Baseplate_V2_v4 (Autodesk Fusion 360 design; units mm, degrees)
Autodesk Fusion 360 part; units mm, degrees
sketch "Esquisse2" plane through (0, 0, 0) normal (0, 0, 1) x (1, 0, 0)
  line L0 (160, 106.25) -> (-160, 106.25)
  line L1 (-160, 106.25) -> (-160, -106.25)
  line L2 (160, -106.25) -> (160, 106.25)
  line L3 (160, 106.25) -> (-160, -106.25) construction
  line L4 (-160, 106.25) -> (160, -106.25) construction
  line L5 (0, 0) -> (65, 0) construction
  line L6 (95, 45) -> (65, 45)
  line L7 (65, 45) -> (65, -45)
  line L8 (65, -45) -> (95, -45)
  line L9 (95, -45) -> (95, 45)
  line L10 (95, 45) -> (65, -45) construction
  line L11 (65, 45) -> (95, -45) construction
  line L12 (110, 45) -> (95, 45)
  line L13 (95, 45) -> (95, -45)
  line L14 (95, -45) -> (110, -45)
  line L15 (110, -45) -> (110, 45)
  line L16 (110, 45) -> (95, -45) construction
  line L17 (95, 45) -> (110, -45) construction
  circle A0 centre (150, 96.25) radius 2.5
  line L18 (0, 2.5) -> (0, 20)
  circle A1 centre (-150, 96.25) radius 2.5
  circle A2 centre (150, -96.25) radius 2.5
  circle A3 centre (-150, -96.25) radius 2.5
  circle A4 centre (0, 86.25) radius 12.5
  circle A5 centre (115, -106.25) radius 12.5
  line L19 (0, 1.75) -> (0, 22.5)
  circle A6 centre (-115, -106.25) radius 12.5
  arc A7 (-131.5, -106.25) -> (-98.5, -106.25) centre (-115, -106.25) ccw
  line L20 (-160, -106.25) -> (-131.5, -106.25)
  arc A8 (98.5, -106.25) -> (131.5, -106.25) centre (115, -106.25) ccw
  line L21 (-98.5, -106.25) -> (98.5, -106.25)
  line L22 (131.5, -106.25) -> (160, -106.25)
  line L23 (-65, 45) -> (-65, -45)
  line L24 (-95, 45) -> (-65, 45)
  line L25 (-110, 45) -> (-95, 45)
  line L26 (-110, -45) -> (-110, 45)
  line L27 (-95, -45) -> (-110, -45)
  line L28 (-65, -45) -> (-95, -45)
  line L29 (-155, 70) -> (-150, 70)
  line L30 (-150, 70) -> (-150, 30)
  line L31 (-150, 30) -> (-155, 30)
  line L32 (-155, 30) -> (-155, 70)
  line L33 (-155, -30) -> (-155, -70)
  line L34 (-150, -30) -> (-155, -30)
  line L35 (-150, -70) -> (-150, -30)
  line L36 (-155, -70) -> (-150, -70)
  line L37 (150, -70) -> (150, -30)
  line L38 (155, -70) -> (150, -70)
  line L39 (155, -30) -> (155, -70)
  line L40 (150, -30) -> (155, -30)
  line L41 (155, 30) -> (155, 70)
  line L42 (155, 70) -> (150, 70)
  line L43 (150, 70) -> (150, 30)
  line L44 (150, 30) -> (155, 30)
  point P0 (80, 0)
  point P1 (102.5, 0)
  dimension "d39" = 212.5
  dimension "d40" = 65
  dimension "d41" = 50
  dimension "d42" = 30
  dimension "d43" = 15
  dimension "d44" = 90
  dimension "d45" = 90
  dimension "d46" = 5
  dimension "d47" = 10
  dimension "d48" = 10
  dimension "d49" = 25
  dimension "d50" = 20
  dimension "d51" = 25
  dimension "d52" = 45
  dimension "d54" = 4
  dimension "d56" = 4
  dimension "d57" = 28.5
  dimension "d58" = 5
  dimension "d59" = 40
  dimension "d60" = 5
  dimension "d61" = 30
  constraint horizontal L0
  constraint perpendicular L0 L1
  constraint parallel L0 L20
  constraint parallel L1 L2
  constraint coincident L3 L5.start
  constraint coincident L4 L5.start
  constraint coincident L5.start origin
  constraint horizontal L5
  constraint horizontal L6
  constraint perpendicular L6 L7
  constraint parallel L6 L8
  constraint parallel L7 L9
  constraint coincident L10 P0
  constraint coincident L11 P0
  constraint horizontal L12
  constraint perpendicular L12 L13
  constraint parallel L12 L14
  constraint parallel L13 L15
  constraint coincident L16 P1
  constraint coincident L17 P1
  constraint collinear L9 L13
  constraint coincident L5.end L7
  constraint coincident L5 P0
  constraint coincident L5 P1
  constraint symmetric A0 L18 A1
  constraint symmetric L5 A0 A2
  constraint symmetric L5 A1 A3
  constraint coincident A5.centre L20
  constraint coincident A4.centre L19
  constraint symmetric A5 L19 A6
  constraint concentric A6 A7
  constraint coincident A7.end L20
  constraint collinear L20 L21
  constraint concentric A5 A8
  constraint coincident A8.end L21
  constraint symmetric L6.start L18 L24.start
  constraint symmetric L6.end L18 L23.start
  constraint symmetric L7.end L18 L23.end
  constraint symmetric L8.end L18 L27.start
  constraint symmetric L12.start L18 L25.start
  constraint symmetric L14.end L18 L26.start
  constraint horizontal L29
  constraint vertical L30
  constraint horizontal L31
  constraint vertical L32
  constraint symmetric L5 L29.start L33.end
  constraint symmetric L5 L29.end L35.start
  constraint symmetric L5 L30.end L34.start
  constraint symmetric L5 L31.end L33.start
  constraint symmetric L19 L29.start L41.end
  constraint symmetric L19 L29.end L42.end
  constraint symmetric L19 L30.end L43.end
  constraint symmetric L19 L31.end L41.start
  constraint symmetric L19 L33.start L39.start
  constraint symmetric L19 L33.end L38.start
  constraint symmetric L19 L34.start L37.end
  constraint symmetric L19 L35.start L37.start
  measures "d39" distance of L0.end L1.end
  measures "d40" distance of L5.start L5.end
  measures "d41" distance of L2 L15
  measures "d42" distance of L6.start L6.end
  measures "d43" distance of L12.start L6.start
  measures "d44" distance of L12.start L14.end
  measures "d45" distance of L6.end L7.end
  measures "d46" diameter of A0
  measures "d47" distance of L2 A0.centre
  measures "d48" distance of L0 A0.centre
  measures "d49" diameter of A4
  measures "d50" distance of L0 A4.centre
  measures "d51" diameter of A5
  measures "d52" distance of L2 A5.centre
  measures "d54" distance of A6 A7
  measures "d56" distance of A5 A8
  measures "d57" distance of L2.start A8.end
  measures "d58" distance of L29.start L29.end
  measures "d59" distance of L29.end L30.end
  measures "d60" distance of L1 L32
  measures "d61" distance of L5 L31
extrude "Extrusion1" add sketch "Esquisse2" along normal blind 3
fillet "Congé1" radius 10 4 edges at (160, -106.25, 1.5) (-160, -106.25, 1.5) (-160, 106.25, 1.5) (160, 106.25, 1.5)
fillet "Congé2" radius 10 4 edges at (131.5, -106.25, 1.5) (98.5, -106.25, 1.5) (-131.5, -106.25, 1.5) (-98.5, -106.25, 1.5)
equation "baseWidth = 250 mm"
equation "baseDepth = ( maxPerimeter - sparePerimeter - 2 * baseWidth ) / 2"
equation "maxPerimeter = ( 2050 / 2 ) * 1 mm"
equation "maxDeployedPerimeter = ( 2200 / 2 ) * 1 mm"
equation "baseRatio = 2 / 3"
equation "sparePerimeter = 100 mm"
equation "baseThickness = 3 mm"
equation "chamferWidth = 30 mm"
equation "motorLength = 65 mm"
equation "wheelHoleWidth = 30 mm"
equation "encoderWheelHoleWidth = 15 mm"
equation "encoderAndSupportWidth = 40 mm"
equation "d39 = baseDepth"
equation "d42 = wheelHoleWidth"
equation "d43 = encoderWheelHoleWidth"
equation "d45 = d44"
equation "d51 = d49"
